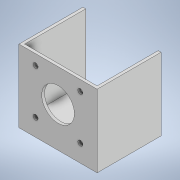
# Autodesk Inventor part: Motorhalterung_v2
Saved by Autodesk Inventor 2021 (Build 250183000, 183)
## iProperties
Created: 2021-01-03
Part Number: Motorhalterung_v2
Material: Generisch
Document SubType Name: Modeling
Designer: Ctroi
Density: 1 g/cm^3
Appearance: Vorgabe
Mass: 18.8981 g
Surface Area: 175.763 cm^2
Volume: 18.8981 cm^3
Author: Ctroi
Autodesk Inventor part; units mm, degrees
ref_plane "YZ Plane" through (0, 0, 0) normal (1, 0, 0) x (0, 1, 0)
ref_plane "XZ Plane" through (0, 0, 0) normal (0, 1, 0) x (-1, 0, 0)
ref_plane "XY Plane" through (0, 0, 0) normal (0, 0, 1) x (1, 0, 0)
sketch "Skizze1" plane through (0, 0, 0) normal (0, 1, 0) x (-1, 0, 0)
  line L0 (-27.5, 22.5) -> (27.5, 22.5)
  line L1 (27.5, 22.5) -> (27.5, -22.5)
  line L2 (27.5, -22.5) -> (-27.5, -22.5)
  line L3 (-27.5, -22.5) -> (-27.5, 22.5)
  line L4 (0, -31.5) -> (0, 31.5) projected
  line L5 (38.5, 0) -> (-38.5, 0) projected
  point P0 (0, 0)
  dimension "d0" = 55
  dimension "d1" = 45
  constraints: 8 end point, 2 parallel, 1 horizontal, 1 perpendicular, 2 other
  measures "d0" distance of L1.end L2.end
  measures "d1" distance of L0.end L1.end
extrude "Extrusion1" add sketch "Skizze1" along normal blind 3
sketch "Skizze2" plane through (0, 3, 0) normal (0, 1, 0) x (1, 0, 0)
  line L0 (-27.5, 22.5) -> (-27.5, -22.5) projected
  line L1 (27.5, -22.5) -> (27.5, 22.5) projected
  line L2 (-27.5, -22.5) -> (27.5, -22.5)
  line L3 (27.5, -22.5) -> (27.5, -20.5)
  line L4 (27.5, -20.5) -> (-27.5, -20.5)
  line L5 (-27.5, -20.5) -> (-27.5, -22.5)
  point P0 (0, 0)
  dimension "d4" = 2
  constraints: 8 end point, 2 parallel, 1 horizontal, 1 perpendicular, 1 point on line
  measures "d4" distance of L3.end L2.end
extrude "Extrusion2" add sketch "Skizze2" along normal blind 45
sketch "Skizze3" plane through (-27.5, 0, 22.5) normal (0, 0, 1) x (1, 0, 0)
  circle A0 centre (27.5, 25) radius 11.5
  line L0 (0, 0) -> (55, 0) projected
  line L1 (55, 0) -> (55, 48) projected
  circle A1 centre (43.25, 9.25) radius 1.75
  circle A2 centre (11.75, 9.25) radius 1.75
  circle A3 centre (11.75, 40.75) radius 1.75
  circle A4 centre (43.25, 40.75) radius 1.75
  line L2 (0, 48) -> (55, 48) projected
  line L3 (27.5, 48) -> (27.5, 0)
  line L4 (4.6208, 25) -> (55, 25)
  dimension "d7" = 23
  dimension "d10" = 3.5
  dimension "d11" = 3.5
  dimension "d12" = 3.5
  dimension "d13" = 3.5
  dimension "d17" = 31.5
  dimension "d48" = 0
  constraints: 5 centre point, 4 end point, 3 symmetric about line, 2 perpendicular, 1 midpoint, 1 point on line
  measures "d7" diameter of A0
  measures "d10" diameter of A1
  measures "d11" diameter of A2
  measures "d12" diameter of A3
  measures "d13" diameter of A4
  measures "d17" diameter of A4.centre L3
  measures "d48" distance from line of A0.centre L3
extrude "Extrusion3" cut sketch "Skizze3" against normal up to surface (2 mm away) contours L4 L3 A0 | A0 L3 L4 | L3 L4 A0 | A0 L4 L3 | A1 | A2 | A3 | A4
sketch "Skizze10" plane through (0, 3, 0) normal (0, 1, 0) x (1, 0, 0)
  line L0 (27.5, -20.5) -> (27.5, 22.5) projected
  line L1 (27.5, 22.5) -> (-27.5, 22.5) projected
  line L2 (27.5, -20.5) -> (25.5, -20.5)
  line L3 (25.5, -20.5) -> (25.5, 22.5)
  line L4 (25.5, 22.5) -> (27.5, 22.5)
  line L5 (27.5, 22.5) -> (27.5, -20.5)
  line L6 (27.5, -20.5) -> (-27.5, -20.5) projected
  line L7 (-27.5, 22.5) -> (-25.5, 22.5)
  line L8 (-25.5, 22.5) -> (-25.5, -20.5)
  line L9 (-25.5, -20.5) -> (-27.5, -20.5)
  line L10 (-27.5, -20.5) -> (-27.5, 22.5)
  point P0 (0, 0)
  point P1 (-27.5, -20.5)
  dimension "d43" = 2
  dimension "d44" = 2
  constraints: 16 end point, 4 parallel, 2 horizontal, 2 perpendicular, 2 point on line
  measures "d43" distance of L3.end L4.end
  measures "d44" distance of L8.end L9.end
extrude "Extrusion6" add sketch "Skizze10" along normal up to surface (45 mm away) contours L2 L3 L1 L0 | L6 L10 L1 L8
sketch "Skizze11" plane through (0, 0, 0) normal (0, -1, 0) x (1, 0, 0)
  line L0 (27.5, 22.5) -> (27.5, -22.5) projected
  line L1 (-27.5, 22.5) -> (27.5, 22.5) projected
  line L2 (27.5, -22.5) -> (-27.5, -22.5)
  line L3 (-27.5, -22.5) -> (-27.5, 22.5)
  line L4 (-27.5, 22.5) -> (27.5, 22.5)
  line L5 (27.5, 22.5) -> (27.5, -22.5)
  point P0 (0, 0)
  constraints: 8 end point, 2 parallel, 1 horizontal, 1 perpendicular
extrude "Extrusion7" add sketch "Skizze11" along normal blind 3
sketch "Skizze12" plane through (25.5, 3, -22.5) normal (0, 0, -1) x (-1, 0, 0)
  line L0 (6, -1.5) -> (14, -1.5)
  line L1 (14, -1.5) -> (14, -4.5)
  line L2 (14, -4.5) -> (6, -4.5)
  line L3 (6, -4.5) -> (6, -1.5)
  line L4 (45, -1.5) -> (37, -1.5)
  line L5 (37, -1.5) -> (37, -4.5)
  line L6 (37, -4.5) -> (45, -4.5)
  line L7 (45, -4.5) -> (45, -1.5)
  line L8 (21.5, -1.5) -> (29.5, -1.5)
  line L9 (29.5, -1.5) -> (29.5, -4.5)
  line L10 (29.5, -4.5) -> (21.5, -4.5)
  line L11 (21.5, -4.5) -> (21.5, -1.5)
  line L12 (0, 0) -> (51, 0) projected
  line L13 (-2, -6) -> (-2, 45) projected
  line L14 (53, 45) -> (53, -6) projected
  point P0 (25.5, -3)
  dimension "d52" = 8
  dimension "d53" = 3
  dimension "d54" = 8
  dimension "d55" = 3
  dimension "d56" = 8
  dimension "d57" = 3
  dimension "d58" = 1.5
  dimension "d59" = 1.5
  dimension "d60" = 1.5
  dimension "d61" = 8
  dimension "d62" = 8
  dimension "d63" = 7.5
  constraints: 24 end point, 6 parallel, 3 horizontal, 3 perpendicular
  measures "d52" distance of L1.end L2.end
  measures "d53" distance of L0.end L1.end
  measures "d54" distance of L6.end L5.end
  measures "d55" distance of L5.end L4.end
  measures "d56" distance of L9.end L10.end
  measures "d57" distance of L8.end L9.end
  measures "d58" distance between parallel lines of L12 L0
  measures "d59" distance between parallel lines of L12 L8
  measures "d60" distance between parallel lines of L12 L4
  measures "d61" distance between parallel lines of L13 L3
  measures "d62" distance between parallel lines of L14 L7
  measures "d63" distance between parallel lines of L11 L1
extrude "Extrusion8" cut sketch "Skizze12" against normal blind 30
